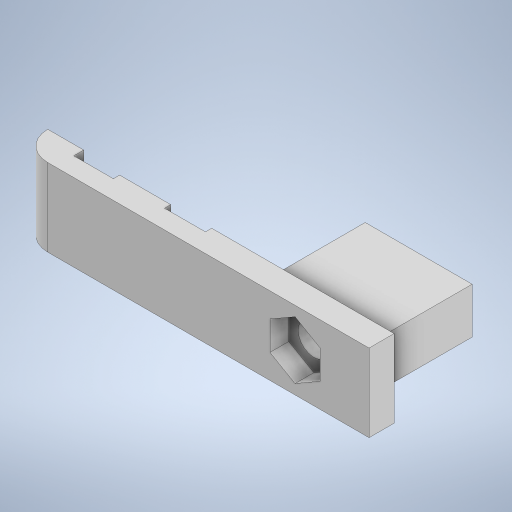
# Autodesk Inventor part: stereotax_side
Saved by Autodesk Inventor 2023.3 (Build 273359000, 359)
## iProperties
Created: 2023-07-12
Part Number: stereotax_side
Material: Generic
Document SubType Name: Modeling
Designer: joao
Density: 1 g/cm^3
Appearance: Default
Author: joao
Autodesk Inventor part; units mm, degrees
ref_plane "YZ Plane" through (0, 0, 0) normal (1, 0, 0) x (0, 1, 0)
ref_plane "XZ Plane" through (0, 0, 0) normal (0, 1, 0) x (-1, 0, 0)
ref_plane "XY Plane" through (0, 0, 0) normal (0, 0, 1) x (1, 0, 0)
sketch "Sketch1" plane through (0, 0, 0) normal (0, 0, 1) x (1, 0, 0)
  line L0 (0.142, 0.105) -> (28.1, 0.105)
  line L1 (28.1, -1.295) -> (0.142, -1.295)
  line L2 (0.142, -1.295) -> (0.142, 0.105)
  line L3 (28.1, -1.295) -> (28.1, 0.105)
  line L4 (0.142, -1.295) -> (0.142, 0.105)
  line L5 (10.2623, 4.905) -> (13.5348, 4.905) projected
  line L6 (6.1805, 3.905) -> (10.2623, 3.905) projected
  line L7 (10.2623, 0.105) -> (6.1805, 0.105) projected
  line L8 (0.142, 4.905) -> (28.1, 4.905)
  line L9 (28.1, 4.905) -> (28.1, 3.905)
  line L10 (28.1, 3.905) -> (0.142, 3.905)
  line L11 (0.142, 3.905) -> (0.142, 4.905)
  line L12 (0.142, -1.295) -> (0.142, 0.105)
  line L13 (28.1, 3.905) -> (28.1, 0.105)
  line L14 (0.142, 3.905) -> (0.142, 0.105)
  line L15 (3.1, -1.295) -> (29.6, -1.295) projected
  line L16 (0.142, -1.295) -> (0.142, 0.105) projected
  constraints: 24 end point, 7 collinear, 4 parallel, 2 horizontal, 1 perpendicular, 1 vertical
extrude "side" add sketch "Sketch1" along normal blind 2
sketch "Sketch2" plane through (0, 0, 0) normal (0, 0, -1) x (-1, 0, 0)
  line L0 (-26.6, -0.295) -> (-17.7228, -0.295) projected
  circle A0 centre (-22.1893, 1.8051) radius 1.1 projected
  line L1 (-26.6, -0.295) -> (-17.7228, -0.295) projected
  line L2 (-26.6, 3.705) -> (-26.6, -0.295) projected
  line L3 (-17.7228, 3.705) -> (-26.6, 3.705) projected
  line L4 (-17.8928, -0.125) -> (-26.43, -0.125)
  line L5 (-26.43, -0.125) -> (-26.43, 3.535)
  line L6 (-26.43, 3.535) -> (-17.8928, 3.535)
  circle A1 centre (-22.1893, 1.8051) radius 1.25
  line L7 (-17.8928, 3.535) -> (-17.8928, -0.125)
  line L8 (-17.7228, -0.295) -> (-17.7228, 3.905) projected
  point P0 (0, 0)
  dimension "d2" = 0.17
  dimension "d4" = 0.17
  dimension "d5" = 0.17
  dimension "d6" = 2.5
  dimension "d25" = 0.17
  constraints: 8 end point, 1 centre point, 1 coincident, 1 horizontal, 1 parallel, 1 perpendicular, 1 vertical, 1 other
  measures "d2" distance between parallel lines of L0 L4
  measures "d5" distance between parallel lines of L2 L5
  measures "d6" diameter of A1
  measures "d25" distance between parallel lines of L8 L7
extrude "sliding_block" add sketch "Sketch2" along normal blind 7.9 contours L4 L5 L6 L7
sketch "Sketch3" plane through (22.1893, 1.8051, 0) normal (0, 0, -1) x (-1, 0, 0)
  circle A0 centre (0, 0) radius 1.25 projected
  point P0 (22.1893, -1.8051)
extrude "hole" cut sketch "Sketch3" against normal up to surface (2 mm away)
sketch "Sketch4" plane through (0, 0, 0) normal (0, 0, -1) x (-1, 0, 0)
  line L0 (-3.0135, 4.905) -> (-6.1805, 4.905) projected
  line L1 (-3.0135, 3.905) -> (-3.0135, 4.905) projected
  line L2 (-0.3963, 3.905) -> (-3.0135, 3.905) projected
  line L3 (-3.0135, 0.105) -> (-0.3963, 0.105) projected
  line L4 (-3.0135, -1.295) -> (-3.0135, 0.105) projected
  line L5 (-6.1805, -1.295) -> (-3.0135, -1.295) projected
  line L6 (-6.1805, 0.105) -> (-6.1805, -1.295) projected
  line L7 (-10.2623, 0.105) -> (-6.1805, 0.105) projected
  line L8 (-10.2623, -1.295) -> (-10.2623, 0.105) projected
  line L9 (-13.5348, -1.295) -> (-10.2623, -1.295) projected
  line L10 (-13.5348, 0.105) -> (-13.5348, -1.295) projected
  line L11 (-14, 0.105) -> (-13.5348, 0.105) projected
  line L12 (-14, 3.905) -> (-14, 0.105) projected
  line L13 (-13.5348, 3.905) -> (-14, 3.905) projected
  line L14 (-13.5348, 4.905) -> (-13.5348, 3.905) projected
  line L15 (-10.2623, 4.905) -> (-13.5348, 4.905) projected
  line L16 (-10.2623, 3.905) -> (-10.2623, 4.905) projected
  line L17 (-6.1805, 3.905) -> (-10.2623, 3.905) projected
  line L18 (-6.1805, 4.905) -> (-6.1805, 3.905) projected
  line L19 (-6.1805, -1.295) -> (-3.0135, -1.295) projected
  line L20 (-6.1805, 0.105) -> (-6.1805, -1.295) projected
  line L21 (-10.2623, 0.105) -> (-6.1805, 0.105) projected
  line L22 (-10.2623, -1.295) -> (-10.2623, 0.105) projected
  line L23 (-13.5348, -1.295) -> (-10.2623, -1.295) projected
  line L24 (-13.5348, 0.105) -> (-13.5348, -1.295) projected
  line L25 (-14, 0.105) -> (-13.5348, 0.105) projected
  line L26 (-14, 3.905) -> (-14, 0.105) projected
  line L27 (-13.5348, 3.905) -> (-14, 3.905) projected
  line L28 (-13.5348, 4.905) -> (-13.5348, 3.905) projected
  line L29 (-10.2623, 4.905) -> (-13.5348, 4.905) projected
  line L30 (-10.2623, 3.905) -> (-10.2623, 4.905) projected
  line L31 (-6.1805, 3.905) -> (-10.2623, 3.905) projected
  line L32 (-6.1805, 4.905) -> (-6.1805, 3.905) projected
  line L33 (-3.0135, 4.905) -> (-6.1805, 4.905) projected
  line L34 (-3.0135, 3.905) -> (-3.0135, 4.905) projected
  line L35 (-0.3963, 3.905) -> (-3.0135, 3.905) projected
  line L36 (-0.3963, 0.105) -> (-0.3963, 3.905) projected
  line L37 (-3.0135, 0.105) -> (-0.3963, 0.105) projected
  line L38 (-3.0135, -1.295) -> (-3.0135, 0.105) projected
  line L39 (-0.3963, 0.105) -> (-0.142, 0.105)
  line L40 (-0.142, 4.905) -> (-0.142, -1.295) projected
  line L41 (-0.3963, 3.905) -> (-0.142, 3.905)
  line L42 (-0.142, 3.905) -> (-0.142, 0.105)
  constraints: 6 end point, 3 point on line, 1 horizontal, 1 perpendicular
extrude "alignment_cut" cut sketch "Sketch4" against normal blind 0.5
sketch "Sketch5" plane through (0, 0, 2) normal (0, 0, 1) x (1, 0, 0)
  line L0 (22.1893, 4.1145) -> (24.1893, 2.9598)
  line L1 (24.1893, 2.9598) -> (24.1893, 0.6504)
  line L2 (24.1893, 0.6504) -> (22.1893, -0.5043)
  line L3 (22.1893, -0.5043) -> (20.1893, 0.6504)
  line L4 (20.1893, 0.6504) -> (20.1893, 2.9598)
  line L5 (20.1893, 2.9598) -> (22.1893, 4.1145)
  circle A0 centre (22.1893, 1.8051) radius 1.25 projected
  point P0 (0, 0)
  dimension "d19" = 4
  constraints: 12 end point, 2 coincident, 1 vertical, 13 other
  measures "d19" distance between parallel lines of L4 L1
sketch "Sketch6" plane through (0, 0, 0) normal (0, 0, -1) x (-1, 0, 0)
  line L0 (-0.142, -1.295) -> (-28.1, -1.295) projected
  line L1 (-0.142, -1.295) -> (-28.1, -1.295) projected
  line L2 (-28.1, 4.905) -> (-0.142, 4.905) projected
  line L3 (-28.1, 4.905) -> (-13.5348, 4.905) projected
  line L4 (-3.0135, 3.905) -> (-3.0135, 4.905) projected
  line L5 (-0.142, 4.905) -> (-3.0135, 4.905) projected
  line L6 (-0.142, 3.905) -> (-3.0135, 3.905) projected
  line L7 (-0.142, -1.295) -> (-3.0135, -1.295) projected
  line L8 (-13.5348, -1.295) -> (-13.5348, 0.105) projected
  line L9 (-13.5348, 0.105) -> (-14, 0.105) projected
  line L10 (-14, 0.105) -> (-14, 3.905) projected
  line L11 (-14, 3.905) -> (-13.5348, 3.905) projected
  line L12 (-13.5348, 3.905) -> (-13.5348, 4.905) projected
  line L13 (-13.5348, -1.295) -> (-28.1, -1.295) projected
  line L14 (-10.2623, 0.105) -> (-10.2623, -1.295) projected
  line L15 (-6.1805, -1.295) -> (-10.2623, -1.295) projected
  line L16 (-6.1805, -1.295) -> (-6.1805, 0.105) projected
  line L17 (-6.1805, 0.105) -> (-10.2623, 0.105) projected
  line L18 (-3.0135, 0.105) -> (-3.0135, -1.295) projected
  line L19 (-0.142, 4.905) -> (-0.142, 3.905) projected
  line L20 (-3.0135, 4.905) -> (-3.0135, 3.905) projected
  line L21 (-10.2623, 4.905) -> (-10.2623, 3.905) projected
  line L22 (-10.2623, 3.905) -> (-6.1805, 3.905) projected
  line L23 (-6.1805, 3.905) -> (-6.1805, 4.905) projected
  line L24 (-3.0135, 4.905) -> (-0.142, 4.905) projected
  line L25 (-10.2623, 4.905) -> (-6.1805, 4.905) projected
  line L26 (-28.1, -1.295) -> (-28.1, 4.905) projected
  line L27 (-26.43, 3.535) -> (-17.8928, 3.535) projected
  line L28 (-17.8928, 3.535) -> (-17.8928, -0.125) projected
  line L29 (-17.8928, -0.125) -> (-26.43, -0.125) projected
  line L30 (-26.43, -0.125) -> (-26.43, 3.535) projected
  line L31 (-0.142, 3.905) -> (-0.142, 4.905) projected
  line L32 (-0.142, 0.105) -> (-0.142, -1.295) projected
  line L33 (-0.142, 0.105) -> (-3.0135, 0.105) projected
  line L34 (-3.0135, 3.905) -> (-0.142, 3.905) projected
  point P0 (-0.1, 0.105)
  point P1 (-0.1, 3.905)
extrude "probe_slot" add sketch "Sketch6" along normal blind 0.3 contours L0 L18 L33 L32 | L2 L19 L6 L4
extrude "nut_slot" cut sketch "Sketch5" against normal blind 1.5 contours L0 L1 L2 L3 L4 L5 | A0
fillet "Fillet3" radius 2.3 1 edges at (0.142, 1.805, 2)
equation "\"d4\" = d2"
equation "\"d5\" = d2"
equation "\"d25\" = d2"
body "Solid1"
